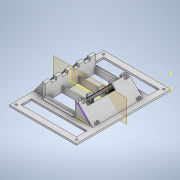
# Autodesk Inventor part: top_casing
Saved by Autodesk Inventor 2020.1 (Build 241239000, 239)
## iProperties
Created: 2019-06-30
Part Number: top_casing
Material: Generic
Document SubType Name: Modeling
Designer: jjsch
Density: 1 g/cm^3
Appearance: Default
Mass: 59.4685 g
Surface Area: 420 cm^2
Volume: 59.4685 cm^3
Author: jjsch
Autodesk Inventor part; units mm, degrees
ref_plane "YZ Plane" through (0, 0, 0) normal (1, 0, 0) x (0, 1, 0)
ref_plane "XZ Plane" through (0, 0, 0) normal (0, 1, 0) x (-1, 0, 0)
ref_plane "XY Plane" through (0, 0, 0) normal (0, 0, 1) x (1, 0, 0)
sketch "Sketch1" plane through (0, 0, 0) normal (0, 1, 0) x (-1, 0, 0)
  line L0 (0, 0) -> (120, 0)
  line L1 (120, 0) -> (120, 168)
  line L2 (120, 168) -> (0, 168)
  line L3 (0, 168) -> (0, 0)
  dimension "d2" = 120
  dimension "d3" = 168
  constraints: 8 end point, 2 parallel, 1 horizontal, 1 perpendicular
  measures "d2" distance of L2.end L1.end
  measures "d3" distance of L1.end L0.end
extrude "Extrusion1" add sketch "Sketch1" along normal blind 3
sketch "Sketch2" plane through (0, 3, 0) normal (0, 1, 0) x (1, 0, 0)
  point P0 (0, 0)
sketch "Sketch3" plane through (0, 3, 0) normal (0, 1, 0) x (1, 0, 0)
  line L0 (-100, -129) -> (-10, -129)
  line L1 (-10, -129) -> (-10, -39)
  line L2 (-10, -39) -> (-100, -39)
  line L3 (-100, -39) -> (-100, -129)
  line L4 (-120, 0) -> (-120, -168) projected
  line L5 (0, -168) -> (0, 0) projected
  line L6 (-120, -168) -> (0, -168) projected
  line L7 (0, 0) -> (-120, 0) projected
  dimension "d6" = 90
  dimension "d7" = 90
  dimension "d8" = 20
  dimension "d9" = 10
  dimension "d10" = 39
  dimension "d11" = 39
  constraints: 8 end point, 2 parallel, 1 horizontal, 1 perpendicular
  measures "d6" distance of L2.end L1.end
  measures "d7" distance of L1.end L0.end
  measures "d8" distance between parallel lines of L4 L3
  measures "d9" distance between parallel lines of L5 L1
  measures "d10" distance between parallel lines of L6 L0
  measures "d11" distance between parallel lines of L7 L2
extrude "Extrusion2" add sketch "Sketch3" along normal blind 40 contours L3 L2 L1 L0
chamfer "Chamfer1" distance 40 angle 45 1 edges at (-10, 43, 84)
sketch "Sketch4" plane through (-50, 43, 39) normal (0.7071068, 0.7071068, 0) x (-0.7071068, 0.7071068, 0)
  circle A0 centre (-22.5685, 82.5) radius 1.5
  circle A1 centre (-22.5685, 7.5) radius 1.5
  circle A2 centre (-53.5685, 7.5) radius 1.5
  circle A3 centre (-53.5685, 82.5) radius 1.5
  line L0 (-56.5685, 0) -> (0, 0) projected
  line L1 (0, 90) -> (-56.5685, 90) projected
  line L2 (-56.5685, 0) -> (-56.5685, 90) projected
  line L3 (-19.5685, 90) -> (-19.5685, 0)
  circle A4 centre (-22.5685, 7.5) radius 2.5
  circle A5 centre (-53.5685, 7.5) radius 2.5
  circle A6 centre (-53.5685, 82.5) radius 2.5
  circle A7 centre (-22.5685, 82.5) radius 2.5
  point P0 (-65.7609, -39)
  point P1 (-16.9706, 0)
  point P2 (-16.9706, 90)
  dimension "d17" = 3
  dimension "d18" = 3
  dimension "d19" = 3
  dimension "d20" = 3
  dimension "d21" = 31
  dimension "d22" = 31
  dimension "d23" = 75
  dimension "d24" = 75
  dimension "d25" = 90
  dimension "d26" = 7.5
  dimension "d27" = 0
  dimension "d28" = 3
  dimension "d29" = 0
  dimension "d30" = 34
  dimension "d31" = 3
  dimension "d37" = 5
  dimension "d38" = 5
  dimension "d39" = 5
  dimension "d40" = 5
  constraints: 8 centre point, 4 coincident, 2 end point, 2 point on line, 1 perpendicular
  measures "d17" diameter of A0
  measures "d18" diameter of A1
  measures "d19" diameter of A2
  measures "d20" diameter of A3
  measures "d21" distance of A3.centre A0.centre
  measures "d22" distance of A1.centre A2.centre
  measures "d23" distance of A3.centre A2.centre
  measures "d24" distance of A0.centre A1.centre
  measures "d25" distance between parallel lines of L0 L1
  measures "d26" distance from line of L0 A2.centre
  measures "d27" vertical distance of A2.centre A1.centre
  measures "d28" distance from line of L2 A3.centre
  measures "d29" horizontal distance of A2.centre A3.centre
  measures "d30" distance from line of A0.centre L2
  measures "d31" distance from line of A0.centre L3
  measures "d37" diameter of A4
  measures "d38" diameter of A5
  measures "d39" diameter of A6
  measures "d40" diameter of A7
sketch "Sketch5" plane through (-100, 3, 129) normal (0, 0, 1) x (1, 0, 0)
  line L0 (0, 0) -> (0, 40) projected
  line L1 (50, 40) -> (90, 0) projected
  line L2 (0, 40) -> (63.8371, 40)
  line L3 (63.8371, 40) -> (63.8371, 26.1629)
  line L4 (63.8371, 26.1629) -> (0, 26.1629)
  line L5 (0, 26.1629) -> (0, 40)
  point P0 (100, -3)
  constraints: 8 end point, 2 parallel, 1 horizontal, 1 perpendicular, 1 point on line
extrude "Extrusion3" cut sketch "Sketch5" against normal blind 300 contours L0 L2 L1 L4
sketch "Sketch8" plane through (-10, 3, 39) normal (0.7071068, 0.7071068, 0) x (-0.7071068, 0.7071068, 0)
  point P0 (-9.1924, -39)
extrude "Extrusion5" add sketch "Sketch4" along normal blind 5 contours A4 | A5 | A6 | A7
sketch "Sketch9" plane through (-10, 3, 39) normal (0.7071068, 0.7071068, 0) x (-0.7071068, 0.7071068, 0)
  point P0 (-9.1924, -39)
sketch "Sketch10" plane through (-10, 3, 39) normal (0.7071068, 0.7071068, 0) x (-0.7071068, 0.7071068, 0)
  point P0 (-9.1924, -39)
sketch "Sketch11" plane through (-100, 29.1629, 129) normal (0, 1, 0) x (1, 0, 0)
  point P0 (100, 129)
sketch "Sketch12" plane through (-100, 29.1629, 129) normal (0, 1, 0) x (1, 0, 0)
  line L0 (58.4186, 0) -> (5.4186, 0)
  line L1 (5.4186, 0) -> (5.4186, 90)
  line L2 (5.4186, 90) -> (58.4186, 90)
  line L3 (58.4186, 90) -> (58.4186, 0)
  line L4 (63.8371, 90) -> (63.8371, 0) projected
  line L5 (0, 0) -> (0, 90) projected
  line L6 (63.8371, 0) -> (0, 0) projected
  point P0 (100, 129)
  dimension "d43" = 53
  dimension "d44" = 5.4185
  dimension "d45" = 5.4186
  dimension "d46" = 0
  dimension "d47" = 90
  constraints: 8 end point, 2 parallel, 1 horizontal, 1 perpendicular
  measures "d43" distance of L0.start L0.end
  measures "d44" distance between parallel lines of L4 L3
  measures "d45" distance between parallel lines of L5 L1
  measures "d46" distance between parallel lines of L6 L0
  measures "d47" distance between parallel lines of L0 L2
extrude "Extrusion6" cut sketch "Sketch12" against normal blind 40
sketch "Sketch13" plane through (-36.1629, 29.1629, 129) normal (0, 1, 0) x (1, 0, 0)
  line L0 (26.1629, 90) -> (0, 90) projected
  line L1 (-5.4185, 0) -> (-5.4185, 90) projected
  line L2 (0, 90) -> (-5.4185, 90)
  line L3 (-5.4185, 90) -> (-5.4185, 80)
  line L4 (-5.4185, 80) -> (0, 80)
  line L5 (0, 80) -> (0, 90)
  line L6 (0, 0) -> (-5.4185, 0) projected
  line L7 (-63.8371, 90) -> (-58.4185, 90) projected
  line L8 (-58.4185, 90) -> (-58.4185, 0) projected
  line L9 (-63.8371, 90) -> (-58.4185, 90)
  line L10 (-58.4185, 90) -> (-58.4185, 80)
  line L11 (-58.4185, 80) -> (-63.8371, 80)
  line L12 (-63.8371, 80) -> (-63.8371, 90)
  line L13 (0, 80) -> (-5.4185, 80)
  line L14 (-5.4185, 80) -> (-5.4185, 70)
  line L15 (-5.4185, 70) -> (0, 70)
  line L16 (0, 70) -> (0, 80)
  line L17 (-63.8371, 80) -> (-58.4185, 80)
  line L18 (-58.4185, 80) -> (-58.4185, 70)
  line L19 (-58.4185, 70) -> (-63.8371, 70)
  line L20 (-63.8371, 70) -> (-63.8371, 80)
  line L21 (0, 70) -> (-5.4185, 70)
  line L22 (-5.4185, 70) -> (-5.4185, 60)
  line L23 (-5.4185, 60) -> (0, 60)
  line L24 (0, 60) -> (0, 70)
  line L25 (-63.8371, 70) -> (-58.4185, 70)
  line L26 (-58.4185, 70) -> (-58.4185, 60)
  line L27 (-58.4185, 60) -> (-63.8371, 60)
  line L28 (-63.8371, 60) -> (-63.8371, 70)
  line L29 (0, 60) -> (-5.4185, 60)
  line L30 (-5.4185, 60) -> (-5.4185, 50)
  line L31 (-5.4185, 50) -> (0, 50)
  line L32 (0, 50) -> (0, 60)
  line L33 (-63.8371, 60) -> (-58.4185, 60)
  line L34 (-58.4185, 60) -> (-58.4185, 50)
  line L35 (-58.4185, 50) -> (-63.8371, 50)
  line L36 (-63.8371, 50) -> (-63.8371, 60)
  line L37 (0, 50) -> (-5.4185, 50)
  line L38 (-5.4185, 50) -> (-5.4185, 40)
  line L39 (-5.4185, 40) -> (0, 40)
  line L40 (0, 40) -> (0, 50)
  line L41 (-63.8371, 50) -> (-58.4185, 50)
  line L42 (-58.4185, 50) -> (-58.4185, 40)
  line L43 (-58.4185, 40) -> (-63.8371, 40)
  line L44 (-63.8371, 40) -> (-63.8371, 50)
  line L45 (0, 40) -> (-5.4185, 40)
  line L46 (-5.4185, 40) -> (-5.4185, 30)
  line L47 (-5.4185, 30) -> (0, 30)
  line L48 (0, 30) -> (0, 40)
  line L49 (-63.8371, 40) -> (-58.4185, 40)
  line L50 (-58.4185, 40) -> (-58.4185, 30)
  line L51 (-58.4185, 30) -> (-63.8371, 30)
  line L52 (-63.8371, 30) -> (-63.8371, 40)
  line L53 (0, 30) -> (-5.4185, 30)
  line L54 (-5.4185, 30) -> (-5.4185, 20)
  line L55 (-5.4185, 20) -> (0, 20)
  line L56 (0, 20) -> (0, 30)
  line L57 (-63.8371, 30) -> (-58.4185, 30)
  line L58 (-58.4185, 30) -> (-58.4185, 20)
  line L59 (-58.4185, 20) -> (-63.8371, 20)
  line L60 (-63.8371, 20) -> (-63.8371, 30)
  line L61 (0, 20) -> (-5.4185, 20)
  line L62 (-5.4185, 20) -> (-5.4185, 10)
  line L63 (-5.4185, 10) -> (0, 10)
  line L64 (0, 10) -> (0, 20)
  line L65 (-63.8371, 20) -> (-58.4185, 20)
  line L66 (-58.4185, 20) -> (-58.4185, 10)
  line L67 (-58.4185, 10) -> (-63.8371, 10)
  line L68 (-63.8371, 10) -> (-63.8371, 20)
  line L69 (0, 10) -> (-5.4185, 10)
  line L70 (-5.4185, 10) -> (-5.4185, 0)
  line L71 (-5.4185, 0) -> (0, 0)
  line L72 (0, 0) -> (0, 10)
  line L73 (-63.8371, 10) -> (-58.4185, 10)
  line L74 (-58.4185, 10) -> (-58.4185, 0)
  line L75 (-58.4185, 0) -> (-63.8371, 0)
  line L76 (-63.8371, 0) -> (-63.8371, 10)
  point P0 (36.1629, 129)
  point P1 (-63.8371, 20)
  point P2 (-58.4185, 10)
  point P3 (-58.4185, 20)
  point P4 (-63.8371, 40)
  point P5 (-58.4185, 30)
  point P6 (-58.4185, 40)
  point P7 (-63.8371, 60)
  point P8 (-58.4185, 50)
  point P9 (-58.4185, 60)
  point P10 (-63.8371, 80)
  point P11 (-58.4185, 70)
  point P12 (0, 80)
  point P13 (-5.4185, 70)
  point P14 (0, 60)
  point P15 (-5.4185, 60)
  point P16 (0, 40)
  point P17 (-5.4185, 40)
  point P18 (-5.4185, 30)
  point P19 (0, 20)
  point P20 (-5.4185, 20)
  point P21 (-5.4185, 10)
  dimension "d50" = 10
  dimension "d51" = 90
  dimension "d52" = 10
  dimension "d55" = 10
  constraints: 144 end point, 4 parallel, 2 horizontal, 2 perpendicular, 2 point on line, 1 vertical, 128 other
  measures "d50" distance of L3.end L2.end
  measures "d51" distance between parallel lines of L6 L2
  measures "d52" distance of L9.end L10.end
  measures "d55" distance of L3.end L14.end
extrude "Extrusion7" cut sketch "Sketch13" against normal blind 5 contours L1 L55 L64 L63 | L1 L39 L48 L47 | L1 L23 L32 L31 | L1 L4 L16 L15 | L11 L8 L19 L20 | L27 L8 L35 L36 | L43 L8 L51 L52 | L59 L8 L67 L68
sketch "Sketch14" plane through (-10, 3, 39) normal (0, 0, -1) x (-1, 0, 0)
  line L0 (31.5814, 0) -> (31.5814, 26.1629) projected
  line L1 (31.5814, 26.1629) -> (26.1629, 26.1629) projected
  line L2 (0, 0) -> (26.1629, 26.1629) projected
  line L3 (31.5814, 0) -> (0, 0) projected
  line L4 (31.5814, 0) -> (31.5814, 26.1629) projected
  line L5 (31.5814, 26.1629) -> (26.1629, 26.1629) projected
  line L6 (0, 0) -> (26.1629, 26.1629) projected
  line L7 (31.5814, 0) -> (0, 0) projected
  line L8 (26.9914, 24.1629) -> (29.5814, 24.1629)
  line L9 (29.5814, 24.1629) -> (29.5814, 2)
  line L10 (29.5814, 2) -> (4.8284, 2)
  line L11 (4.8284, 2) -> (26.9914, 24.1629)
  point P0 (-10, -3)
  dimension "d62" = 2
  constraints: 8 end point, 3 other
  measures "d62" distance between parallel lines of L2 L11
extrude "Extrusion8" cut sketch "Sketch14" against normal through all contours L8 L9 L10 L11
sketch "Sketch15" plane through (-14.8284, 5, 39) normal (-0.7071068, -0.7071068, 0) x (0.7071068, -0.7071068, 0)
  line L0 (-31.3431, 0) -> (-33.1746, 0) projected
  line L1 (-31.3431, 0) -> (0, 0)
  line L2 (0, 0) -> (0, 90.1505)
  line L3 (0, 90.1505) -> (-31.3431, 90.1505)
  line L4 (-31.3431, 90.1505) -> (-31.3431, 0)
  point P0 (14.0208, -39)
  constraints: 8 end point, 2 parallel, 1 horizontal, 1 perpendicular
sketch "Sketch17" plane through (-39.5814, 27.1629, 69) normal (0, -1, 0) x (1, 0, 0)
  point P0 (39.5814, -69)
sketch "Sketch18" plane through (-39.5814, 5, 129) normal (0, 1, 0) x (1, 0, 0)
  point P0 (39.5814, 129)
sketch "Sketch19" plane through (-39.5814, 5, 39) normal (0, 1, 0) x (1, 0, 0)
  line L0 (2.5901, -90.1505) -> (2.5901, 0) projected
  line L1 (24.753, -90) -> (0, -90) projected
  line L2 (24.753, 0) -> (24.753, -90) projected
  line L3 (0, 0) -> (24.753, 0) projected
  line L4 (0, 0) -> (0, -90) projected
  line L5 (3.4185, -10) -> (3.4185, -20) projected
  point P0 (39.5814, 39)
sketch "Sketch20" plane through (-41.5814, 3, 129) normal (0, 0, 1) x (1, 0, 0)
  line L0 (26.753, 2) -> (2, 2) projected
  line L1 (2, 2) -> (2, 24.1629) projected
  line L2 (2, 24.1629) -> (4.5901, 24.1629) projected
  line L3 (4.5901, 24.1629) -> (26.753, 2) projected
  line L4 (0, 26.1629) -> (0, 0) projected
  line L5 (31.5814, 0) -> (0, 0) projected
  line L6 (5.4185, 26.1629) -> (31.5814, 0) projected
  line L7 (5.4185, 26.1629) -> (0, 26.1629) projected
  point P0 (41.5814, -3)
extrude "Extrusion10" add sketch "Sketch20" against normal up to surface (10 mm away) contours L0 L1 L2 L3
sketch "Sketch21" plane through (-10, 3, 39) normal (0, 0, -1) x (-1, 0, 0)
  line L0 (29.5814, 2) -> (4.8284, 2) projected
  line L1 (4.8284, 2) -> (26.9914, 24.1629) projected
  line L2 (26.9914, 24.1629) -> (29.5814, 24.1629) projected
  line L3 (29.5814, 24.1629) -> (29.5814, 2) projected
  line L4 (31.5814, 0) -> (31.5814, 26.1629) projected
  line L5 (31.5814, 26.1629) -> (26.1629, 26.1629) projected
  line L6 (0, 0) -> (26.1629, 26.1629) projected
  line L7 (31.5814, 0) -> (0, 0) projected
  point P0 (-10, -3)
extrude "Extrusion11" add sketch "Sketch21" against normal up to surface (10 mm away) contours L0 L1 L2 L3
sketch "Sketch22" plane through (-10, 3, 39) normal (0.7071068, 0.7071068, 0) x (-0.7071068, 0.7071068, 0)
  line L0 (37, 80) -> (37, 90) projected
  line L1 (37, 80) -> (27, 80)
  line L2 (27, 80) -> (27, 30)
  line L3 (27, 30) -> (37, 30)
  line L4 (37, 30) -> (37, 80)
  point P0 (-9.1924, -39)
  dimension "d80" = 10
  dimension "d81" = 50
  constraints: 8 end point, 2 parallel, 1 horizontal, 1 perpendicular
  measures "d80" distance of L3.end L2.end
  measures "d81" distance of L2.end L1.end
extrude "Extrusion12" cut sketch "Sketch22" against normal up to surface surface through (-39.5814, 27.1629, 39) normal (-1, 0, 0)
sketch "Sketch23" plane through (-41.5814, 29.1629, 69) normal (0, 0, 1) x (1, 0, 0)
  line L0 (0, 0) -> (5.4185, 0) projected
  line L1 (2, -2) -> (5.4185, -2)
  line L2 (5.4185, -2) -> (5.4185, 0)
  line L3 (5.4185, 0) -> (2, 0)
  line L4 (2, 0) -> (2, -2)
  point P0 (41.5814, -29.1629)
  constraints: 8 end point, 2 parallel, 1 horizontal, 1 perpendicular
extrude "Extrusion13" cut sketch "Sketch23" along normal blind 20 and the other way blind 50
sketch "Sketch24" plane through (-41.5814, 24.1629, 99) normal (0, 0, -1) x (-1, 0, 0)
  line L0 (-2, 3) -> (-5.8371, 3)
  line L1 (-5.8371, 3) -> (-5.8371, 6.1897)
  line L2 (-5.8371, 6.1897) -> (-2, 6.1897)
  line L3 (-2, 6.1897) -> (-2, 3)
  point P0 (-41.5814, -24.1629)
  constraints: 8 end point, 2 parallel, 1 horizontal, 1 perpendicular
extrude "Extrusion14" cut sketch "Sketch24" against normal up to surface (20 mm away)
sketch "Sketch26" plane through (0, 3, 0) normal (0, 1, 0) x (1, 0, 0)
  line L0 (-100, -39) -> (-94.5814, -39) projected
  line L1 (-94.5814, -39) -> (-41.5814, -39) projected
  line L2 (-41.5814, -39) -> (-10, -39) projected
  line L3 (-10, -39) -> (-10, -129) projected
  line L4 (-10, -129) -> (-41.5814, -129) projected
  line L5 (-41.5814, -129) -> (-94.5814, -129) projected
  line L6 (-94.5814, -129) -> (-100, -129) projected
  line L7 (-100, -129) -> (-100, -39) projected
  line L8 (-120, 0) -> (-120, -168) projected
  line L9 (-120, -168) -> (0, -168) projected
  line L10 (0, -168) -> (0, 0) projected
  line L11 (0, 0) -> (-120, 0) projected
  line L12 (-114, -6) -> (-114, -162)
  line L13 (-114, -162) -> (-6, -162)
  line L14 (-6, -162) -> (-6, -6)
  line L15 (-6, -6) -> (-114, -6)
  dimension "d92" = 6
  dimension "d100" = 6
  constraints: 8 end point, 4 coincident, 3 other
  measures "d92" distance between parallel lines of L11 L15
  measures "d100" distance between parallel lines of L8 L12
hole "Hole1" at (-114, 3, 162) at (-114, 3, 6) at (-6, 3, 162) at (-6, 3, 6) direction (0, -1, 0) diameter 4 end through all
sketch "Sketch27" plane through (0, 3, 0) normal (0, 1, 0) x (1, 0, 0)
  line L0 (-100, -129) -> (-100, -119) projected
  line L1 (-100, -124) -> (-120, -124)
  line L2 (-120, 0) -> (-120, -168) projected
  line L3 (-100, -124) -> (-80, -124) construction
  line L4 (-100, -129) -> (-100, -39) projected
  line L5 (-120, -123.25) -> (-100, -123.25)
  line L6 (-100, -123.25) -> (-100, -124.75)
  line L7 (-100, -124.75) -> (-120, -124.75)
  line L8 (-120, -124.75) -> (-120, -123.25)
  line L9 (-120, -123.25) -> (-100, -124.75) construction
  line L10 (-100, -123.25) -> (-120, -124.75) construction
  line L11 (-100, -104) -> (-120, -104)
  line L12 (-120, -103.25) -> (-100, -103.25)
  line L13 (-100, -103.25) -> (-100, -104.75)
  line L14 (-100, -104.75) -> (-120, -104.75)
  line L15 (-120, -104.75) -> (-120, -103.25)
  line L16 (-120, -103.25) -> (-100, -104.75) construction
  line L17 (-100, -103.25) -> (-120, -104.75) construction
  line L18 (-100, -84) -> (-120, -84)
  line L19 (-120, -83.25) -> (-100, -83.25)
  line L20 (-100, -83.25) -> (-100, -84.75)
  line L21 (-100, -84.75) -> (-120, -84.75)
  line L22 (-120, -84.75) -> (-120, -83.25)
  line L23 (-120, -83.25) -> (-100, -84.75) construction
  line L24 (-100, -83.25) -> (-120, -84.75) construction
  line L25 (-100, -64) -> (-120, -64)
  line L26 (-120, -63.25) -> (-100, -63.25)
  line L27 (-100, -63.25) -> (-100, -64.75)
  line L28 (-100, -64.75) -> (-120, -64.75)
  line L29 (-120, -64.75) -> (-120, -63.25)
  line L30 (-120, -63.25) -> (-100, -64.75) construction
  line L31 (-100, -63.25) -> (-120, -64.75) construction
  line L32 (-100, -44) -> (-120, -44)
  line L33 (-120, -43.25) -> (-100, -43.25)
  line L34 (-100, -43.25) -> (-100, -44.75)
  line L35 (-100, -44.75) -> (-120, -44.75)
  line L36 (-120, -44.75) -> (-120, -43.25)
  line L37 (-120, -43.25) -> (-100, -44.75) construction
  line L38 (-100, -43.25) -> (-120, -44.75) construction
  point P0 (0, 0)
  point P1 (-110, -124)
  point P2 (-110, -104)
  point P3 (-110, -84)
  point P4 (-110, -64)
  point P5 (-110, -44)
  dimension "d101" = 180
  dimension "d102" = 5
  dimension "d103" = 5
  dimension "d104" = 1.5
  dimension "d107" = 20
  constraints: 72 end point, 15 midpoint, 2 horizontal, 2 parallel, 2 point on line, 1 collinear, 1 perpendicular, 1 vertical, 56 other
  measures "d101" angle of L1 L3
  measures "d102" distance from line of L0.start L1
  measures "d103" distance of L1.start L0.end
  measures "d104" distance of L5.end L6.end
  measures "d107" distance of L1.start L11.start
extrude "Extrusion16" add sketch "Sketch27" along normal up to surface (26.1629 mm away) contours L7 L2 L1 L0 | L1 L2 L5 L0 | L14 L2 L11 L4 | L11 L2 L12 L4 | L21 L2 L18 L4 | L18 L2 L19 L4 | L28 L2 L25 L4 | L25 L2 L26 L4 | L35 L2 L32 L4 | L32 L2 L33 L4
chamfer "Chamfer2" distance 20 distance2 26.613 1 edges at (-120, 29.1629, 124) measured on face at (-119.5, 29.1629, 124)
sketch "Sketch28" plane through (-36.9914, 27.1629, 69) normal (0, 1, 0) x (1, 0, 0)
  line L0 (0.8284, 0) -> (0, 0) projected
  line L1 (0.8284, 10) -> (0.8284, 0) projected
  line L2 (0, 10) -> (0.8284, 10) projected
  line L3 (0, 10) -> (0, 0) projected
  point P0 (36.9914, 69)
extrude "Extrusion17" cut sketch "Sketch28" against normal blind 5
sketch "Sketch29" plane through (-39.5814, 27.1629, 49) normal (0, 1, 0) x (1, 0, 0)
  line L0 (3.4185, 0) -> (0, 0) projected
  line L1 (3.4185, 10) -> (3.4185, 0) projected
  line L2 (0, 10) -> (3.4185, 10) projected
  line L3 (0, 0) -> (0, 10) projected
  point P0 (39.5814, 49)
extrude "Extrusion18" cut sketch "Sketch29" against normal blind 3
ref_plane "Work Plane1" through (-10, 3, 84) normal (0, 0, -1) x (-1, 0, 0)
mirror "Mirror1" about plane through (-10, 3, 84) normal (0, 0, -1) of "Extrusion18"
sketch "Sketch30" plane through (-39.5814, 24.1629, 119) normal (0, 1, 0) x (1, 0, 0)
  line L0 (3.4185, -10) -> (3.4185, 0) projected
  line L1 (0, 0) -> (3.4185, 0) projected
  line L2 (0, 0) -> (0, -10) projected
  line L3 (3.4185, -10) -> (0, -10) projected
  point P0 (39.5814, 119)
extrude "Extrusion19" cut sketch "Sketch30" along normal blind 5
sketch "Sketch31" plane through (-94.5814, 3, 129) normal (1, 0, 0) x (0, 0, -1)
  point P0 (129, -3)
sketch "Sketch32" plane through (-94.5814, 3, 129) normal (1, 0, 0) x (0, 0, -1)
  line L0 (90, -3) -> (88, -3)
  line L1 (88, -3) -> (88, 7.543)
  line L2 (88, 7.543) -> (90, 7.543)
  line L3 (90, 7.543) -> (90, -3)
  point P0 (129, -3)
  dimension "d123" = 2
  dimension "d124" = 10.543
  constraints: 8 end point, 2 parallel, 1 horizontal, 1 perpendicular
  measures "d123" distance of L1.end L2.end
  measures "d124" distance of L0.end L1.end
extrude "Extrusion20" add sketch "Sketch32" along normal up to next
pattern_linear "Rectangular Pattern1" count 4 spacing 29.3333 along (0, 0, 1) of "Extrusion20"
ref_plane "Work Plane2" through (-120, 0, 84) normal (0, 0, 1) x (1, 0, 0)
sketch "Sketch36" plane through (-120, 0, 84) normal (0, 0, 1) x (1, 0, 0)
  line L0 (25.4186, 10.543) -> (78.4186, 10.543) projected
  line L1 (25.4186, 10.543) -> (25.4186, 29.1629) projected
  point P0 (120, 0)
sketch "Sketch37" plane through (-100, 3, 129) normal (0, 0, 1) x (1, 0, 0)
  line L0 (5.4186, 7.543) -> (5.4186, 26.1629) projected
  line L1 (5.4186, 7.543) -> (58.4186, 7.543) projected
  line L2 (58.4186, 26.1629) -> (58.4186, 7.543) projected
  line L3 (0, 0) -> (0, 26.1629) projected
  line L4 (5.4186, 7.543) -> (5.4186, -3) projected
  line L5 (58.4186, -3) -> (58.4186, 7.543) projected
  line L6 (5.4186, 5.3909) -> (58.4186, 5.3909)
  line L7 (58.4186, 5.3909) -> (58.4186, 2.3909)
  line L8 (58.4186, 2.3909) -> (5.4186, 2.3909)
  line L9 (5.4186, 2.3909) -> (5.4186, 5.3909)
  point P0 (100, -3)
  point P1 (5.4186, 2.3909)
  dimension "d138" = 3
  constraints: 8 end point, 2 parallel, 2 point on line, 1 horizontal, 1 perpendicular
  measures "d138" distance of L6.end L7.end
extrude "Extrusion23" add sketch "Sketch37" along normal blind 4 contours L6 L5 L8 L4
chamfer "Chamfer4" distance 2 angle 45 1 edges at (-68.0814, 8.3909, 133)
mirror "Mirror2" about plane through (-120, 0, 84) normal (0, 0, 1) of "Extrusion23", "Chamfer4"
sketch "Sketch38" plane through (-100, 3, 129) normal (0, 0, 1) x (1, 0, 0)
  line L0 (5.4186, 5.3909) -> (5.4186, 3.3909) projected
  line L1 (5.4186, 3.3909) -> (58.4186, 3.3909) projected
  line L2 (58.4186, 3.3909) -> (58.4186, 5.3909) projected
  line L3 (58.4186, 5.3909) -> (5.4186, 5.3909) projected
  line L4 (58.4186, 5.3909) -> (5.4186, 5.3909) projected
  line L5 (5.4186, 7.543) -> (58.4186, 7.543) projected
  line L6 (58.4186, 5.3909) -> (5.4186, 5.3909)
  line L7 (5.4186, 5.3909) -> (5.4186, 7.543)
  line L8 (5.4186, 7.543) -> (58.4186, 7.543)
  line L9 (58.4186, 7.543) -> (58.4186, 5.3909)
  point P0 (100, -3)
  constraints: 8 end point, 2 parallel, 1 horizontal, 1 perpendicular
extrude "Extrusion24" add sketch "Sketch38" along normal blind 2 contours L7 L5 L9 L3
mirror "Mirror3" about plane through (-120, 0, 84) normal (0, 0, 1) of "Extrusion24"
sketch "Sketch40" plane through (-41.5814, 29.1629, 119) normal (-1, 0, 0) x (0, 0, 1)
  line L0 (-50.6667, -18.6199) -> (-48.6667, -18.6199) projected
  line L1 (-21.3333, -18.6199) -> (-21.3333, -29.1629)
  line L2 (0, -5) -> (0, -24.1629) projected
  line L3 (-70, -24.1629) -> (0, -24.1629) projected
  line L4 (-70, -24.1629) -> (-70, -5) projected
  line L5 (-60, -5) -> (-70, -5) projected
  line L6 (-60, 0) -> (-60, -5) projected
  line L7 (-50, 0) -> (-60, 0) projected
  line L8 (-50, -5) -> (-50, 0) projected
  line L9 (-40, -5) -> (-50, -5) projected
  line L10 (-40, 0) -> (-40, -5) projected
  line L11 (-30, 0) -> (-40, 0) projected
  line L12 (-30, -5) -> (-30, 0) projected
  line L13 (-20, -5) -> (-30, -5) projected
  line L14 (-20, 0) -> (-20, -5) projected
  line L15 (-10, 0) -> (-20, 0) projected
  line L16 (-10, -5) -> (-10, 0) projected
  line L17 (0, -5) -> (-10, -5) projected
  line L18 (-21.3333, -29.1629) -> (-21.3333, -18.6199) projected
  line L19 (-21.3333, -24.1629) -> (-48.6667, -24.1629)
  line L20 (-48.6667, -24.1629) -> (-48.6667, -11.1629)
  line L21 (-48.6667, -11.1629) -> (-21.3333, -11.1629)
  line L22 (-21.3333, -11.1629) -> (-21.3333, -24.1629)
  line L23 (-19.3333, -18.6199) -> (-19.3333, -29.1629) projected
  line L24 (0, -5) -> (0, -24.1629) projected
  line L25 (-19.3333, -23.8914) -> (0, -23.8914)
  line L26 (0, -23.8914) -> (0, -11.1629)
  line L27 (0, -11.1629) -> (-19.3333, -11.1629)
  line L28 (-19.3333, -11.1629) -> (-19.3333, -23.8914)
  point P0 (-119, -29.1629)
  point P1 (8, -18.6199)
  point P2 (-48.6667, -24.1629)
  point P3 (0, -11.1629)
  dimension "d157" = 13
  dimension "d160" = 0
  constraints: 18 end point, 4 parallel, 3 point on line, 2 horizontal, 2 perpendicular, 1 midpoint
  measures "d157" distance of L19.end L20.end
  measures "d160" distance between parallel lines of L21 L27
extrude "Extrusion26" cut sketch "Sketch40" against normal blind 2 contours L1 L3 L20 L21 L22 | L23 L28 L27 L2 L25
sketch "Sketch41" plane through (0, 3, 0) normal (0, 1, 0) x (1, 0, 0)
  line L0 (-10, -39) -> (-10, -129) projected
  line L1 (-10, -129) -> (-100, -129) projected
  line L2 (-100, -129) -> (-100, -124.75) projected
  line L3 (-100, -124.75) -> (-119.6618, -124.75) projected
  line L4 (-119.6618, -168) -> (-119.6618, -124.75) projected
  line L5 (-119.6618, -168) -> (0, -168) projected
  line L6 (0, -168) -> (0, 0) projected
  line L7 (0, 0) -> (-119.6618, 0) projected
  line L8 (-119.6618, -43.25) -> (-119.6618, 0) projected
  line L9 (-119.6618, -43.25) -> (-100, -43.25) projected
  line L10 (-100, -43.25) -> (-100, -39) projected
  line L11 (-100, -39) -> (-10, -39) projected
  circle A0 centre (-114, -6) radius 4.2 projected
  line L12 (-109.6618, -139) -> (0, -139)
  line L13 (0, -139) -> (0, -29)
  line L14 (0, -29) -> (-109.6618, -29)
  line L15 (-109.6618, -29) -> (-109.6618, -10)
  line L16 (-109.6618, -10) -> (-10, -10)
  line L17 (-10, -10) -> (-10, -158)
  line L18 (-10, -158) -> (-109.6618, -158)
  line L19 (-109.6618, -158) -> (-109.6618, -139)
  point P0 (-10, -29)
  point P1 (-10, -139)
  dimension "d167" = 10
  constraints: 16 end point, 7 other
  measures "d167" distance between parallel lines of L4 L19
extrude "Extrusion27" cut sketch "Sketch41" against normal blind 10 contours L14 L15 L16 L17 | L17 L18 L19 L12
sketch "Sketch42" plane through (-41.5814, 5.3909, 129) normal (1, 0, 0) x (0, 0, -1)
  line L0 (94, 1) -> (92, 3) projected
  line L1 (92, 3) -> (92, 5.1521) projected
  line L2 (94, 1) -> (92, 3) projected
  line L3 (92, 3) -> (92, 5.1521) projected
  line L4 (90, 5.1521) -> (92, 5.1521) projected
  line L5 (90, 0) -> (90, 5.1521) projected
  line L6 (90, 0) -> (94, 0) projected
  line L7 (94, 0) -> (94, 1) projected
  line L8 (-4, 1) -> (-2, 3) projected
  line L9 (-4, 0) -> (-4, 1) projected
  line L10 (0, 0) -> (-4, 0) projected
  line L11 (0, 5.1521) -> (0, 0) projected
  line L12 (0, 5.1521) -> (-2, 5.1521) projected
  line L13 (-2, 3) -> (-2, 5.1521) projected
  line L14 (-1.95, 5.1021) -> (-0.05, 5.1021)
  line L15 (-0.05, 5.1021) -> (-0.05, 0.05)
  line L16 (-0.05, 0.05) -> (-3.95, 0.05)
  line L17 (-3.95, 0.05) -> (-3.95, 0.9793)
  line L18 (-3.95, 0.9793) -> (-1.95, 2.9793)
  line L19 (-1.95, 2.9793) -> (-1.95, 5.1021)
  line L20 (91.75, 4.9021) -> (91.75, 2.8964)
  line L21 (91.75, 2.8964) -> (93.75, 0.8964)
  line L22 (93.75, 0.8964) -> (93.75, 0.25)
  line L23 (93.75, 0.25) -> (90.25, 0.25)
  line L24 (90.25, 0.25) -> (90.25, 4.9021)
  line L25 (90.25, 4.9021) -> (91.75, 4.9021)
  point P0 (129, -5.3909)
  point P1 (94, 1)
  dimension "d170" = 0.05
  dimension "d171" = 0.25
  constraints: 24 end point, 10 other
  measures "d170" distance between parallel lines of L12 L14
  measures "d171" distance between parallel lines of L4 L25
extrude "Extrusion28" cut sketch "Sketch42" against normal up to surface (58.4186 mm away)
body "Solid1"
